Autodesk Inventor part; units mm, degrees
(part 2 of 2)
extrude "Extrusion98" add sketch "Sketch107" against normal blind 10
sketch "Sketch108" plane through (0, 0, 50) normal (0, 0, 1) x (1, 0, 0)
  line L0 (11, -49.7965) -> (28.75, -49.7965) projected
  line L1 (11, 49.7965) -> (28.75, 49.7965) projected
  line L2 (11, -49.7965) -> (12, -49.7965)
  line L3 (12, -49.7965) -> (12, 49.7965)
  line L4 (12, 49.7965) -> (11, 49.7965)
  line L5 (11, 49.7965) -> (11, -49.7965)
  point P0 (0, 0)
  dimension "d436" = 1
  constraints: 8 end point, 2 parallel, 1 horizontal, 1 perpendicular, 1 point on line
  measures "d436" distance between parallel lines of L3 L5
extrude "Extrusion99" cut sketch "Sketch108" along normal through all
sketch "Sketch109" plane through (0, 0, 50) normal (0, 0, 1) x (1, 0, 0)
  circle A0 centre (21.6375, -42.2965) radius 2.5 projected
  circle A1 centre (21.6375, 42.2965) radius 2.5 projected
  circle A2 centre (21.6375, 42.2965) radius 13.5
  circle A3 centre (21.6375, -42.2965) radius 13.5
  line L0 (12, 9.56) -> (12, 30.7965) projected
  line L1 (12, -30.7965) -> (12, -9.56) projected
  line L2 (21.6375, 28.7965) -> (12, 28.7965)
  line L3 (12, 28.7965) -> (21.6375, 28.7965)
  line L4 (21.6375, 28.7965) -> (21.6375, 30.7965)
  line L5 (21.6375, 30.7965) -> (12, 30.7965)
  line L6 (12, 30.7965) -> (12, 28.7965)
  line L7 (21.6375, -28.7965) -> (12, -28.7965)
  line L8 (12, -28.7965) -> (12, -30.7965)
  line L9 (12, -30.7965) -> (21.6375, -30.7965)
  line L10 (21.6375, -30.7965) -> (21.6375, -28.7965)
  point P0 (0, 0)
  dimension "d439" = 27
  dimension "d440" = 27
  constraints: 18 end point, 4 parallel, 3 horizontal, 3 perpendicular, 3 vertical alignment, 2 coincident, 1 point on line, 4 other
extrude "Extrusion100" cut sketch "Sketch109" along normal blind 20 contours A0 | A1 | L4 L5 A2 | L2 L0 L5 A2 | A2 L5 L4 | A3 L9 L10 | L10 L9 A3 | A3 L9 L1 L7
sketch "Sketch110" plane through (0, 45.7965, 35) normal (0, 0, -1) x (-1, 0, 0)
  circle A0 centre (0, 0) radius 2.5 projected
  circle A1 centre (-39.6609, -68.6947) radius 2.5 projected
  point P0 (0, -45.7965)
extrude "Extrusion101" add sketch "Sketch110" along normal blind 55
sketch "Sketch111" plane through (0, 0, 15) normal (0, 0, -1) x (-1, 0, 0)
  circle A0 centre (0, 0) radius 9.56 construction
  line L0 (38.5, 12.5) -> (38.5, -19.5) construction
  line L1 (38.5, -19.5) -> (21.5, -19.5) construction
  line L2 (21.5, -19.5) -> (21.5, 12.5) construction
  line L3 (21.5, 12.5) -> (23.7028, 21.1109) construction
  arc A1 (34.085, 24.556) -> (23.7028, 21.1109) centre (30, 19.5) ccw construction
  line L4 (24.1312, 41.7965) -> (34.085, 24.556) construction
  line L5 (-24.1312, 41.7965) -> (24.1312, 41.7965) construction
  line L6 (-37.5759, 18.5096) -> (-24.1312, 41.7965) construction
  arc A2 (-37.5759, -18.5096) -> (-37.5759, 18.5096) centre (-30, 0) ccw construction
  line L7 (-24.1312, -41.7965) -> (-37.5759, -18.5096) construction
  line L8 (24.1312, -41.7965) -> (-24.1312, -41.7965) construction
  line L9 (25.8632, -38.7965) -> (24.1312, -41.7965) construction
  line L10 (25.8632, -38.7965) -> (35.1009, -38.7965) construction
  line L11 (49.5346, -13.7965) -> (35.1009, -38.7965) construction
  line L12 (40.297, -13.7965) -> (49.5346, -13.7965) construction
  line L13 (48.2624, 0) -> (40.297, -13.7965) construction
  line L14 (36.4748, 20.4167) -> (48.2624, 0) construction
  line L15 (36.4748, 20.4167) -> (38.5, 12.5) construction
  line L16 (21.5, 12.5) -> (14.3584, 24.8695)
  line L17 (14.3584, 24.8695) -> (-33.904, 24.8695)
  line L18 (21.5, -12.5) -> (21.5, 12.5) projected
  arc A3 (36.2972, 21.1109) -> (23.7028, 21.1109) centre (30, 19.5) ccw projected
  line L19 (24.1312, 41.7965) -> (-24.1312, 41.7965)
  line L20 (-33.904, 24.8695) -> (-24.1312, 41.7965)
  line L21 (23.7028, 21.1109) -> (21.5, 12.5) projected
  line L22 (21.5, 12.5) -> (41.0455, 12.5)
  line L23 (41.0455, 12.5) -> (24.1312, 41.7965)
  dimension "d445" = 16.9269
  dimension "d446" = 16.9269
  constraints: 12 end point, 2 horizontal, 2 point on line, 1 parallel, 1 perpendicular
  measures "d445" distance between parallel lines of L4 L16
  measures "d446" distance between parallel lines of L5 L17
extrude "Extrusion102" cut sketch "Sketch111" against normal blind 20
sketch "Sketch112" plane through (0, 0, -20) normal (0, 0, -1) x (-1, 0, 0)
  arc A0 (-37.5759, -18.5096) -> (-37.5759, 18.5096) centre (-30, 0) ccw projected
  circle A1 centre (-30, 0) radius 21.5
  point P0 (0, 0)
  dimension "d449" = 43
  constraints: 1 centre point, 1 coincident
  measures "d449" diameter of A1
extrude "Extrusion103" cut sketch "Sketch112" against normal through all
sketch "Sketch113" plane through (0, 0, 36.3) normal (0, 0, 1) x (1, 0, 0)
  arc A0 (12, 11.758) -> (12, -11.758) centre (30, 0) ccw projected
  circle A1 centre (0, 0) radius 8.0625 projected
  line L0 (8.6458, 2.5) -> (7.6651, 2.5)
  line L1 (7.6651, 2.5) -> (7.6651, -2.5)
  line L2 (7.6651, -2.5) -> (8.6458, -2.5)
  line L3 (8.6458, -2.5) -> (8.6458, 2.5)
  point P0 (7.6651, 0)
  dimension "d452" = 5
  constraints: 8 end point, 2 parallel, 1 horizontal, 1 horizontal alignment, 1 midpoint, 1 perpendicular, 1 point on circle, 2 other
  measures "d452" distance of L2.end L0.start
extrude "Extrusion104" cut sketch "Sketch113" along normal through all contours L3 A0 | A0 L2 A1 L0 | A1 L1 picked at (7.7384, -0.5607)
sketch "Sketch114" plane through (21.6375, 42.2965, 75) normal (0, 0, 1) x (1, 0, 0)
  circle A0 centre (0, 0) radius 2.5 projected
  circle A1 centre (0, 0) radius 6.5 projected
  circle A2 centre (0, -84.5929) radius 2.5 projected
  circle A3 centre (0, -84.5929) radius 6.5 projected
  point P0 (-21.6375, -42.2965)
extrude "Extrusion105" cut sketch "Sketch114" against normal blind 1
sketch "Sketch117" plane through (0, 0, 50) normal (0, 0, 1) x (1, 0, 0)
  line L0 (8.6458, -2.5) -> (7.6651, -2.5) projected
  arc A0 (7.6651, 2.5) -> (7.6651, -2.5) centre (0, 0) ccw projected
  line L1 (7.6651, 2.5) -> (8.6458, 2.5) projected
  arc A1 (12, 11.758) -> (8.6458, 2.5) centre (30, 0) ccw projected
  line L2 (12, 11.758) -> (12, 28.7965) projected
  line L3 (12, 28.7965) -> (21.6375, 28.7965) projected
  arc A2 (21.6375, 28.7965) -> (34.8034, 39.3117) centre (21.6375, 42.2965) ccw projected
  line L4 (28.75, 49.7965) -> (34.8034, 39.3117) projected
  line L5 (-28.75, 49.7965) -> (28.75, 49.7965) projected
  line L6 (-57.5, 0) -> (-28.75, 49.7965) construction
  line L7 (-28.75, -49.7965) -> (-57.5, 0) construction
  line L8 (28.75, -49.7965) -> (-28.75, -49.7965) projected
  line L9 (34.8034, -39.3117) -> (28.75, -49.7965) projected
  arc A3 (34.8034, -39.3117) -> (21.6375, -28.7965) centre (21.6375, -42.2965) ccw projected
  line L10 (12, -28.7965) -> (21.6375, -28.7965) projected
  line L11 (12, -28.7965) -> (12, -11.758) projected
  arc A4 (8.6458, -2.5) -> (12, -11.758) centre (30, 0) ccw projected
  line L12 (-38.5, -19.5) -> (-38.5, -12.5) projected
  line L13 (-21.5, -12.5) -> (-38.5, -12.5) projected
  line L14 (-21.5, -12.5) -> (-21.5, -19.5) projected
  line L15 (-21.5, -19.5) -> (-38.5, -19.5) projected
  circle A5 centre (-30, 0) radius 10 projected
  arc A6 (-23.7028, 21.1109) -> (-36.2972, 21.1109) centre (-30, 19.5) ccw projected
  line L16 (-23.7028, 21.1109) -> (-21.5, 12.5) projected
  line L17 (-21.5, 12.5) -> (-38.5, 12.5) projected
  line L18 (-38.5, 12.5) -> (-36.2972, 21.1109) projected
  arc A7 (23.5117, 43.9509) -> (24.0976, 42.7414) centre (21.6375, 42.2965) ccw projected
  arc A8 (23.5117, 43.9509) -> (24.0976, 42.7414) centre (25.5, 44.1673) ccw projected
  arc A9 (24.0976, -42.7414) -> (23.5117, -43.9509) centre (21.6375, -42.2965) ccw projected
  arc A10 (24.0976, -42.7414) -> (23.5117, -43.9509) centre (25.5, -44.1673) ccw projected
  line L19 (12, 28.7965) -> (12, 49.7965)
  line L20 (-28.75, 49.7965) -> (28.75, 49.7965) projected
  line L21 (12, 49.7965) -> (28.75, 49.7965)
  line L22 (12, -28.7965) -> (12, -49.7965)
  line L23 (28.75, -49.7965) -> (-28.75, -49.7965) projected
  line L24 (12, -49.7965) -> (28.75, -49.7965)
  constraints: 8 end point, 3 point on line, 2 collinear, 1 perpendicular
extrude "Extrusion106" add sketch "Sketch117" along normal blind 30 contours L19 L5 L4 A2 L3 | L8 L22 L10 A3 L9 | A8 A7 | A10 A9
sketch "Sketch118" plane through (-39.6609, 22.8982, 35) normal (0, 0, -1) x (-1, 0, 0)
  circle A0 centre (0, 0) radius 2.5 projected
  circle A1 centre (-79.3218, 0) radius 2.5 projected
  circle A2 centre (-39.6609, -68.6947) radius 2.5 projected
  point P0 (-39.6609, -22.8982)
extrude "Extrusion107" add sketch "Sketch118" along normal blind 55
sketch "Sketch119" plane through (0, 0, -20) normal (0, 0, -1) x (-1, 0, 0)
  line L0 (40.326, 26.7463) -> (36.4288, 24.4963)
  line L1 (36.4288, 24.4963) -> (39.4288, 19.3002)
  line L2 (39.4288, 19.3002) -> (43.326, 21.5502)
  line L3 (43.326, 21.5502) -> (40.326, 26.7463)
  line L4 (57.5, 0) -> (28.75, 49.7965) projected
  line L5 (41.826, 24.1482) -> (43.125, 24.8982)
  line L6 (-36.4288, 24.4963) -> (-40.326, 26.7463)
  line L7 (-40.326, 26.7463) -> (-43.326, 21.5502)
  line L8 (-43.326, 21.5502) -> (-39.4288, 19.3002)
  line L9 (-39.4288, 19.3002) -> (-36.4288, 24.4963)
  line L10 (-3, -43.7965) -> (-3, -48.2965)
  line L11 (-3, -48.2965) -> (3, -48.2965)
  line L12 (3, -48.2965) -> (3, -43.7965)
  line L13 (3, -43.7965) -> (-3, -43.7965)
  point P0 (0, 0)
  point P1 (-41.826, 24.1482)
  point P2 (0, -48.2965)
  dimension "d465" = 4.5
  dimension "d466" = 1.5
  dimension "d467" = 6
  dimension "d470" = 360
  constraints: 26 end point, 3 perpendicular, 2 midpoint, 2 parallel, 28 other
  measures "d465" distance of L1.end L2.end
  measures "d466" distance of L5.start L5.end
  measures "d467" distance of L2.end L0.start
extrude "Extrusion108" cut sketch "Sketch119" against normal blind 6
sketch "Sketch120" plane through (0, 0, -14) normal (0, 0, -1) x (-1, 0, 0)
  line L0 (36.4288, 24.4963) -> (40.326, 26.7463) projected
  line L1 (39.4288, 19.3002) -> (36.4288, 24.4963) projected
  line L2 (43.326, 21.5502) -> (39.4288, 19.3002) projected
  line L3 (40.326, 26.7463) -> (43.326, 21.5502) projected
  line L4 (40.326, 26.7463) -> (43.326, 21.5502) projected
  line L5 (57.5, 0) -> (28.75, 49.7965) projected
  line L6 (40.326, 26.7463) -> (41.625, 27.4963)
  line L7 (41.625, 27.4963) -> (44.625, 22.3002)
  line L8 (44.625, 22.3002) -> (43.326, 21.5502)
  line L9 (43.326, 21.5502) -> (40.326, 26.7463)
  line L10 (-43.326, 21.5502) -> (-44.625, 22.3002)
  line L11 (-44.625, 22.3002) -> (-41.625, 27.4963)
  line L12 (-40.326, 26.7463) -> (-43.326, 21.5502)
  line L13 (-41.625, 27.4963) -> (-40.326, 26.7463)
  line L14 (3, -48.2965) -> (3, -49.7965)
  line L15 (3, -49.7965) -> (-3, -49.7965)
  line L16 (-3, -48.2965) -> (3, -48.2965)
  line L17 (-3, -49.7965) -> (-3, -48.2965)
  point P0 (0, 0)
  dimension "d476" = 360
  constraints: 24 end point, 2 parallel, 1 perpendicular, 1 point on line, 25 other
extrude "Extrusion109" cut sketch "Sketch120" along normal blind 3
chamfer "Chamfer1" distance 1 angle 45 3 edges at (0, -48.2965, -20) (-41.826, 24.1482, -20) (41.826, 24.1482, -20)
sketch "Sketch121" plane through (0, 0, 15) normal (0, 0, -1) x (-1, 0, 0)
  arc A0 (-36.4147, -20.5207) -> (-8.8191, -3.6902) centre (-30, 0) ccw projected
  line L0 (-24.1312, -41.7965) -> (-36.4147, -20.5207) projected
  line L1 (24.1312, -41.7965) -> (-24.1312, -41.7965) construction
  line L2 (25.8632, -38.7965) -> (24.1312, -41.7965) projected
  line L3 (25.8632, -38.7965) -> (35.1009, -38.7965) projected
  line L4 (49.5346, -13.7965) -> (35.1009, -38.7965) projected
  line L5 (40.297, -13.7965) -> (49.5346, -13.7965) projected
  line L6 (48.2624, 0) -> (40.297, -13.7965) projected
  line L7 (41.0455, 12.5) -> (48.2624, 0) projected
  line L8 (41.0455, 12.5) -> (38.5, 12.5) projected
  line L9 (38.5, 12.5) -> (38.5, -19.5) projected
  line L10 (38.5, -19.5) -> (21.5, -19.5) projected
  line L11 (21.5, -19.5) -> (21.5, 12.5) projected
  line L12 (21.5, 12.5) -> (14.3584, 24.8695) projected
  line L13 (14.3584, 24.8695) -> (-33.904, 24.8695) projected
  line L14 (-36.4147, 20.5207) -> (-33.904, 24.8695) projected
  arc A1 (-8.8191, 3.6902) -> (-36.4147, 20.5207) centre (-30, 0) ccw projected
  arc A2 (-8.8191, -3.6902) -> (-8.8191, 3.6902) centre (0, 0) ccw projected
  line L15 (25.8632, -38.7965) -> (40.297, -13.7965)
  line L16 (40.297, -13.7965) -> (49.5346, -13.7965)
  line L17 (35.1009, -38.7965) -> (49.5346, -13.7965)
  line L18 (28.75, -49.7965) -> (57.5, 0) projected
  line L19 (25.8632, -38.7965) -> (35.1009, -38.7965)
  constraints: 8 end point, 3 collinear
extrude "Extrusion110" cut sketch "Sketch121" along normal blind 20 contours L15 L10 L9 L5 L4 L3 | L15 L9 L10
extrude "Extrusion111" add sketch "Sketch121" along normal blind 5 contours L15 L10 L9 L5 L4 L3 | L15 L9 L10
sketch "Sketch122" plane through (0, 0, 50) normal (0, 0, -1) x (-1, 0, 0)
  arc A0 (-24.0976, 42.7414) -> (-23.5117, 43.9509) centre (-21.6375, 42.2965) ccw projected
  arc A1 (-24.0976, 42.7414) -> (-23.5117, 43.9509) centre (-25.5, 44.1673) ccw projected
  arc A2 (-23.5117, -43.9509) -> (-24.0976, -42.7414) centre (-25.5, -44.1673) ccw projected
  arc A3 (-23.5117, -43.9509) -> (-24.0976, -42.7414) centre (-21.6375, -42.2965) ccw projected
  point P0 (0, 0)
extrude "Extrusion112" add sketch "Sketch122" along normal blind 35
sketch "Sketch123" plane through (0, 0, 35) normal (0, 0, -1) x (-1, 0, 0)
  line L0 (-24.087, 41.7965) -> (-19.188, 41.7965) projected
  arc A0 (-24.087, 41.7965) -> (-19.188, 41.7965) centre (-21.6375, 42.2965) ccw projected
  point P0 (0, 0)
extrude "Extrusion113" cut sketch "Sketch123" along normal through all
ref_plane "Work Plane4" through (0, 0, 10) normal (0, 0, -1) x (-1, 0, 0)
sketch "Sketch125" plane through (0, 0, 10) normal (0, 0, -1) x (-1, 0, 0)
  arc A0 (-51.4107, 1.9574) -> (-51.4107, -1.9574) centre (-30, 0) ccw projected
  arc A1 (-51.4107, 1.9574) -> (-51.4107, -1.9574) centre (-30, 0) ccw projected
  arc A2 (-51.4107, 1.9574) -> (-51.4107, -1.9574) centre (-51, 0) ccw projected
  circle A3 centre (-51, 0) radius 2
  circle A4 centre (-51, 0) radius 4
  point P0 (0, 0)
  dimension "d495" = 8
  constraints: 2 coincident, 1 centre point, 3 other
  measures "d495" diameter of A4
extrude "Extrusion115" add sketch "Sketch125" along normal blind 30
body "Solid2"
